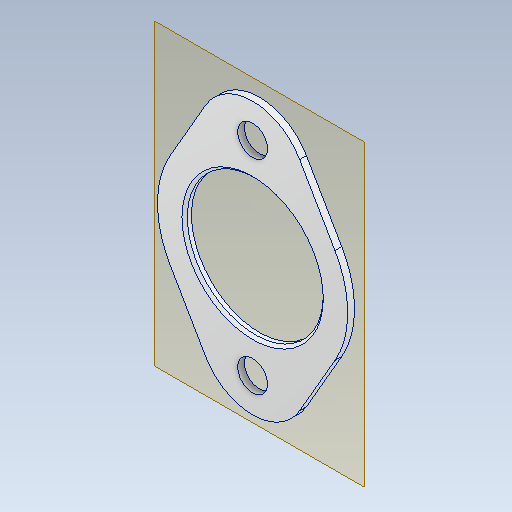
# Autodesk Inventor part: Прокладка крейцкопф_CPY
Saved by Autodesk Inventor 2021 (Build 250183000, 183)
## iProperties
Created: 2020-12-02
Part Number: Прокладка крейцкопф_CPY
Material: Алюминий 6061
Document SubType Name: Modeling
Designer: Тимоха
Mass: 155.66 g
Surface Area: 276.361 cm^2
Volume: 57.652 cm^3
Density: 2.7 g/cm^3
Appearance: Алюминий — плоский
Author: Тимоха
Autodesk Inventor part; units mm, degrees
ref_plane "YZ Plane" through (0, 0, 0) normal (1, 0, 0) x (0, 1, 0)
ref_plane "XZ Plane" through (0, 0, 0) normal (0, 1, 0) x (-1, 0, 0)
ref_plane "XY Plane" through (0, 0, 0) normal (0, 0, 1) x (1, 0, 0)
ref_plane "РабПлоскость1" through (0, 0, 0) normal (0, 0, 1) x (1, 0, 0)
sketch "Эскиз1" plane through (0, 0, 0) normal (0, 0, 1) x (1, 0, 0)
  circle A0 centre (0, 75) radius 8 projected
  circle A1 centre (0, -75) radius 8 projected
  line L0 (34.641, -80) -> (60.6218, -35) projected
  arc A2 (60.6218, -35) -> (60.6218, 35) centre (0, 0) ccw projected
  line L1 (60.6218, 35) -> (34.641, 80) projected
  arc A3 (34.641, 80) -> (-34.641, 80) centre (0, 60) ccw projected
  line L2 (-34.641, 80) -> (-60.6218, 35) projected
  arc A4 (-60.6218, 35) -> (-60.6218, -35) centre (0, 0) ccw projected
  line L3 (-60.6218, -35) -> (-34.641, -80) projected
  arc A5 (-34.641, -80) -> (34.641, -80) centre (0, -60) ccw projected
  circle A6 centre (0, 0) radius 50 projected
  circle A7 centre (0, 75) radius 11
  circle A8 centre (0, -75) radius 11
  point P0 (0, 0)
  dimension "d5" = 22
  dimension "d6" = 16
  dimension "d7" = 22
  constraints: 2 centre point, 2 coincident
  measures "d5" diameter of A7
  measures "d6" diameter of A1
  measures "d7" diameter of A8
extrude "Выдавливание1" add sketch "Эскиз1" along normal blind 5 contours A5 L3 A4 L2 A3 L1 A2 L0
chamfer "Фаска1" distance 2 angle 45 1 edges at (-50, 0, 5)
